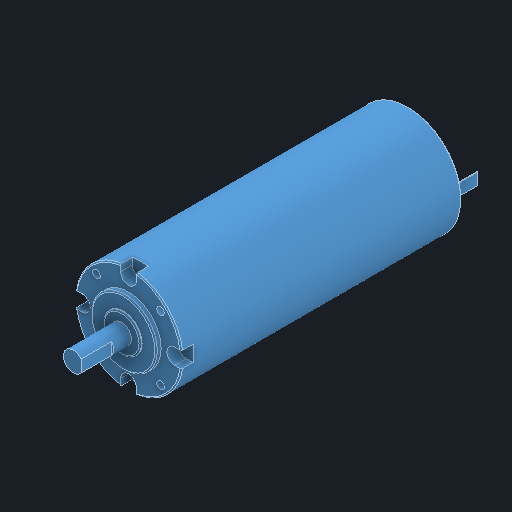
# Autodesk Inventor part: motor
Saved by Autodesk Inventor 2024 (Build 280153000, 153)
## iProperties
Created: 2023-04-14
Part Number: motor
Material: Типовые
Document SubType Name: Modeling
Designer: user
Density: 1 g/cm^3
Appearance: По умолчанию
Author: user
Autodesk Inventor part; units mm, degrees
ref_plane "YZ Plane" through (0, 0, 0) normal (1, 0, 0) x (0, 1, 0)
ref_plane "XZ Plane" through (0, 0, 0) normal (0, 1, 0) x (-1, 0, 0)
ref_plane "XY Plane" through (0, 0, 0) normal (0, 0, 1) x (1, 0, 0)
sketch "Эскиз1" plane through (0, 0, 0) normal (0, 0, 1) x (1, 0, 0)
  circle A0 centre (0, 0) radius 21
  dimension "d0" = 42
  constraints: 1 centre point, 1 coincident
  measures "d0" diameter of A0
extrude "Выдавливание1" add sketch "Эскиз1" along normal blind 110
sketch "Эскиз2" plane through (0, 0, 110) normal (0, 0, 1) x (1, 0, 0)
  circle A0 centre (0, 0) radius 12.85
  dimension "d3" = 25.7
  constraints: 1 centre point, 1 coincident
  measures "d3" diameter of A0
extrude "Выдавливание2" add sketch "Эскиз2" along normal blind 2
sketch "Эскиз3" plane through (0, 0, 110) normal (0, 0, 1) x (1, 0, 0)
  circle A0 centre (0, 0) radius 21 projected
  line L0 (20.7699, 3.1) -> (18.1699, 3.1)
  line L1 (20.7699, -3.1) -> (18.1699, -3.1)
  arc A1 (18.1699, 3.1) -> (18.1699, -3.1) centre (18.1699, 0) ccw
  arc A2 (20.7699, -3.1) -> (20.7699, 3.1) centre (0, 0) ccw
  point P0 (15.0699, 0)
  dimension "d6" = 6.2
  dimension "d7" = 5.7
  constraints: 7 point on circle, 4 end point, 2 centre point, 2 horizontal, 2 tangent, 1 coincident, 1 concentric, 1 horizontal alignment
  measures "d6" distance from line of L1 L0.start
  measures "d7" horizontal distance of L0.start point (15.07, 0)
extrude "Выдавливание3" cut sketch "Эскиз3" against normal blind 4.6 contours A0 L1 A1 L0 picked at (17.0617, 0)
pattern_circular "Круговой массив1" count 4 over 360 about axis through (0, 0, 0) along (0, 0, 1) of "Выдавливание3"
sketch "Эскиз4" plane through (0, 0, 110) normal (0, 0, 1) x (1, 0, 0)
  circle A0 centre (12.5865, 12.5865) radius 1.5
  arc A1 (18.1699, 3.1) -> (18.1699, -3.1) centre (18.1699, 0) ccw construction
  line L0 (18.1699, 0) -> (12.5865, 12.5865) construction
  arc A2 (-3.1, 18.1699) -> (3.1, 18.1699) centre (0, 18.1699) ccw construction
  line L1 (12.5865, 12.5865) -> (0, 18.1699) construction
  line L2 (12.5865, 12.5865) -> (14.8492, 14.8492) construction
  circle A3 centre (0, 0) radius 21 construction
  dimension "d13" = 3
  dimension "d14" = 3.2
  constraints: 6 end point, 1 centre point, 1 equal length, 3 other
  measures "d13" diameter of A0
  measures "d14" distance of L0.end L2.end
extrude "Выдавливание4" cut sketch "Эскиз4" against normal blind 7
pattern_circular "Круговой массив2" count 4 over 360 about axis through (0, 0, 0) along (0, 0, 1) of "Выдавливание4"
sketch "Эскиз5" plane through (0, 0, 112) normal (0, 0, 1) x (1, 0, 0)
  circle A0 centre (0, 0) radius 7.35
  dimension "d20" = 14.7
  constraints: 1 centre point, 1 coincident
  measures "d20" diameter of A0
extrude "Выдавливание5" add sketch "Эскиз5" along normal blind 0.7
sketch "Эскиз6" plane through (0, 0, 112.7) normal (0, 0, 1) x (1, 0, 0)
  circle A0 centre (0, 0) radius 3.9
  dimension "d23" = 7.8
  constraints: 1 centre point, 1 coincident
  measures "d23" diameter of A0
extrude "Выдавливание6" add sketch "Эскиз6" along normal blind 19
sketch "Эскиз7" plane through (0, 0, 131.7) normal (0, 0, 1) x (1, 0, 0)
  circle A0 centre (0, 0) radius 3.9 projected
  line L0 (3.1, -2.3664) -> (3.1, 2.3664)
  arc A1 (3.1, -2.3664) -> (3.1, 2.3664) centre (0, 0) ccw
  line L1 (3.1, 0) -> (-3.9, 0) construction
  dimension "d26" = 7
  constraints: 5 point on circle, 4 end point, 1 centre point, 1 coincident, 1 concentric, 1 horizontal, 1 midpoint, 1 vertical
  measures "d26" distance of L1.start L1.end
extrude "Выдавливание7" cut sketch "Эскиз7" against normal blind 12 contours A0 L0 picked at (3.3667, 0)
sketch "Эскиз8" plane through (0, 0, 0) normal (0, 0, -1) x (-1, 0, 0)
  circle A0 centre (0, 0) radius 13.75
  dimension "d29" = 27.5
  constraints: 1 centre point, 1 coincident
  measures "d29" diameter of A0
extrude "Выдавливание8" add sketch "Эскиз8" along normal blind 1.2
sketch "Эскиз9" plane through (0, 0, -1.2) normal (0, 0, -1) x (-1, 0, 0)
  circle A0 centre (0, 0) radius 21 projected
  circle A1 centre (0, 0) radius 7.25
  dimension "d32" = 14.5
  constraints: 1 centre point, 1 coincident
  measures "d32" diameter of A1
extrude "Выдавливание9" add sketch "Эскиз9" along normal blind 3.7 contours A1
sketch "Эскиз10" plane through (0, 0, -4.9) normal (0, 0, -1) x (-1, 0, 0)
  arc A0 (-3.1, -2.3664) -> (-3.1, 2.3664) centre (0, 0) ccw projected
  circle A1 centre (0, 0) radius 2.35
  dimension "d35" = 4.7
  constraints: 1 centre point, 1 coincident
  measures "d35" diameter of A1
extrude "Выдавливание10" add sketch "Эскиз10" along normal blind 7
sketch "Эскиз11" plane through (0, 0, 0) normal (0, 0, -1) x (-1, 0, 0)
  line L0 (-17.3, -2.3) -> (-17, -2.3)
  line L1 (-17.3, -2.3) -> (-17, -2.3)
  line L2 (-17, -2.3) -> (-17, 2.3)
  line L3 (-17, 2.3) -> (-17.3, 2.3)
  line L4 (-17.3, 2.3) -> (-17.3, -2.3)
  line L5 (17, 2.3) -> (17.3, 2.3)
  line L6 (17.3, 2.3) -> (17.3, -2.3)
  line L7 (17.3, -2.3) -> (17, -2.3)
  line L8 (17, -2.3) -> (17, 2.3)
  point P0 (0, 0)
  point P1 (-17, 0)
  point P2 (17, 0)
  dimension "d38" = 17
  dimension "d39" = 17
  dimension "d41" = 4.6
  dimension "d42" = 0.3
  constraints: 18 end point, 4 parallel, 2 equal length, 2 horizontal, 2 horizontal alignment, 2 midpoint, 2 perpendicular
  measures "d38" horizontal distance of L0.end point (0, 0)
  measures "d39" horizontal distance of L7.end point (0, 0)
  measures "d41" distance of L5.end L6.end
  measures "d42" distance of L5.start L5.end
extrude "Выдавливание11" add sketch "Эскиз11" along normal blind 10
fillet "Сопряжение1" radius 0.5 9 edges at (7.25, 0, -4.9) (13.75, 0, -1.2) (-21, 0, 0) (-14.8492, -14.8492, 110) (14.8492, -14.8492, 110) (-14.8492, 14.8492, 110) (14.8492, 14.8492, 110) (-12.85, 0, 112) (-7.35, 0, 112.7)
chamfer "Фаска1" distance 0.5 angle 45 1 edges at (2.35, 0, -11.9)
